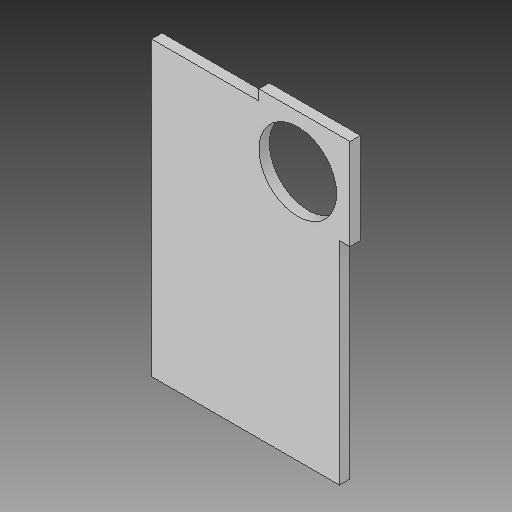
# Autodesk Inventor part: saw blade axle support (hole for arbor)
Saved by Autodesk Inventor 2019 (Build 230136000, 136)
## iProperties
Created: 2018-01-22
Part Number: saw blade axle support (hole for arbor)
Material: Generic
Document SubType Name: Modeling
Designer: Administrator
Density: 1 g/cm^3
Appearance: Default
Author: Administrator
Autodesk Inventor part; units mm, degrees
ref_plane "YZ Plane" through (0, 0, 0) normal (1, 0, 0) x (0, 1, 0)
ref_plane "XZ Plane" through (0, 0, 0) normal (0, 1, 0) x (-1, 0, 0)
ref_plane "XY Plane" through (0, 0, 0) normal (0, 0, 1) x (1, 0, 0)
sketch "Sketch1" plane through (0, 0, 0) normal (0, 0, 1) x (1, 0, 0)
  line L0 (0, 0) -> (114.3, 0)
  line L1 (114.3, 0) -> (114.3, 128.778)
  line L2 (65.278, 177.8) -> (0, 177.8)
  line L3 (0, 177.8) -> (0, 0)
  circle A0 centre (88.9, 152.4) radius 23.622
  line L4 (65.278, 177.8) -> (65.278, 184.15)
  line L5 (65.278, 184.15) -> (120.65, 184.15)
  line L6 (120.65, 184.15) -> (120.65, 128.778)
  line L7 (120.65, 128.778) -> (114.3, 128.778)
  line L8 (120.65, 128.778) -> (114.3, 128.778)
  dimension "d0" = 114.3
  dimension "d2" = 47.244
  dimension "d3" = 25.4
  dimension "d4" = 25.4
  dimension "d5" = 6.35
  dimension "d6" = 6.35
  dimension "d7" = 55.372
  constraints: 18 end point, 5 perpendicular, 2 parallel, 1 centre point, 1 horizontal, 1 vertical
  measures "d0" distance of L0.start L0.end
  measures "d2" diameter of A0
  measures "d3" distance from line of L1 A0.centre
  measures "d4" distance from line of A0.centre L2
  measures "d5" distance between parallel lines of L1 L6
  measures "d6" distance between parallel lines of L2 L5
  measures "d7" distance of L5.end L6.end
extrude "Extrusion1" add sketch "Sketch1" along normal blind 6.35
body "Solid1"
